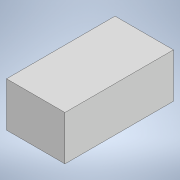
# Autodesk Inventor part: Supongamos_que_es_un_Servo
Saved by Autodesk Inventor 2021 (Build 250183000, 183)
## iProperties
Created: 2020-12-12
Part Number: Supongamos_que_es_un_Servo
Material: Genérico
Document SubType Name: Modeling
Designer: Joaquín
Density: 1 g/cm^3
Appearance: Valor por defecto
Author: Joaquín
Autodesk Inventor part; units mm, degrees
ref_plane "YZ Plane" through (0, 0, 0) normal (1, 0, 0) x (0, 1, 0)
ref_plane "XZ Plane" through (0, 0, 0) normal (0, 1, 0) x (-1, 0, 0)
ref_plane "XY Plane" through (0, 0, 0) normal (0, 0, 1) x (1, 0, 0)
sketch "Boceto1" plane through (0, 0, 0) normal (0, 1, 0) x (-1, 0, 0)
  line L0 (0, 0) -> (21, 0)
  line L1 (21, 0) -> (21, -39)
  line L2 (21, -39) -> (0, -39)
  line L3 (0, -39) -> (0, 0)
  dimension "d3" = 21
  dimension "d4" = 39
  constraints: 8 end point, 3 perpendicular, 1 horizontal
  measures "d3" distance of L0.start L0.end
  measures "d4" distance of L0.end L1.end
extrude "Extrusión1" add sketch "Boceto1" along normal blind 16
